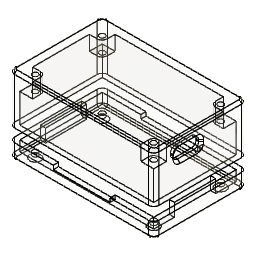
enclosure (Autodesk Fusion 360 design; units mm, degrees)
Autodesk Fusion 360 part; units mm, degrees
sketch "Sketch1" plane through (0, 0, 0) normal (0, 0, 1) x (1, 0, 0) in component "Enclosure-Bottom"
  line L0 (0, 0) -> (50, 0) construction
  line L1 (50, 0) -> (50, 30) construction
  line L2 (50, 30) -> (0, 30) construction
  line L3 (0, 30) -> (0, 0) construction
  line L4 (-1, -1) -> (51, -1)
  line L5 (51, -1) -> (51, 31)
  line L6 (51, 31) -> (-1, 31)
  line L7 (-1, 31) -> (-1, -1)
  line L8 (-1, -3) -> (51, -3)
  line L9 (53, -1) -> (53, 31)
  line L10 (51, 33) -> (-1, 33)
  line L11 (-3, 31) -> (-3, -1)
  arc A0 (53, 31) -> (51, 33) centre (51, 31) ccw
  arc A1 (-1, 33) -> (-3, 31) centre (-1, 31) ccw
  arc A2 (-3, -1) -> (-1, -3) centre (-1, -1) ccw
  arc A3 (51, -3) -> (53, -1) centre (51, -1) ccw
  dimension "d1" = 50
  dimension "d2" = 30
  dimension "d5" = 1
  dimension "d9" = 2
  dimension "d23" = 3
  dimension "d25" = 3
  dimension "d26" = 3
  dimension "d27" = 3
  constraint horizontal L0
  constraint vertical L1
  constraint horizontal L2
  constraint vertical L3
  constraint coincident L0.start L3.end
  constraint parallel L0 L8
  constraint parallel L1 L9
  constraint parallel L2 L10
  constraint parallel L3 L11
  constraint tangent L9 A0
  constraint tangent L10 A0
  constraint tangent L10 A1
  constraint tangent L11 A1
  constraint equal A0 A1
  constraint tangent L11 A2
  constraint tangent L8 A2
  constraint equal A0 A2
  constraint tangent L8 A3
  constraint tangent L9 A3
  constraint equal A0 A3
  measures "d1" distance of L1.end L2.end
  measures "d2" distance of L0.end L1.end
  measures "d9" radius of A0
  measures "d23" distance of L2 L10
  measures "d25" distance of L0 L8
  measures "d26" distance of L3 L11
  measures "d27" distance of L1 L9
extrude "Extrude1" add sketch "Sketch1" against normal blind 2 contours L4 L5 L6 L7 | L8 L9 L10 L11 A0 A1 A2 A3 makes body 1 in component "Enclosure-Bottom"
extrude "Extrude2" add sketch "Sketch1" along normal blind 4 bodies 1 in component "Enclosure-Bottom"
ref_plane "WorkPlane1" through (25, 15, 26) normal (0, 0, 1) x (1, 0, 0)
sketch "Sketch1 (2)" plane through (22.5, 15, 26) normal (0, 0, 1) x (1, 0, 0) in component "Enclosure-Top"
  line L0 (-23.5, -16) -> (28.5, -16)
  line L1 (-23.5, 16) -> (-23.5, -16)
  line L2 (28.5, 16) -> (-23.5, 16)
  line L3 (28.5, -16) -> (28.5, 16)
  line L4 (-23.5, -18) -> (28.5, -18)
  arc A0 (28.5, -18) -> (30.5, -16) centre (28.5, -16) ccw
  line L5 (30.5, -16) -> (30.5, 16)
  line L6 (-25.5, 16) -> (-25.5, -16)
  arc A1 (-25.5, -16) -> (-23.5, -18) centre (-23.5, -16) ccw
  line L7 (28.5, 18) -> (-23.5, 18)
  arc A2 (-23.5, 18) -> (-25.5, 16) centre (-23.5, 16) ccw
  arc A3 (30.5, 16) -> (28.5, 18) centre (28.5, 16) ccw
extrude "Extrude1'" add sketch "Sketch1 (2)" against normal blind 17 separate body makes body 2 in component "Enclosure-Top"
extrude "Extrude2'" add sketch "Sketch1 (2)" along normal blind 2 contours L0 L1 L2 L3 | L4 A0 L5 L6 A1 L7 A2 A3 bodies 2 in component "Enclosure-Top"
fillet "Fillet1" radius 1 8 edges at (53, 15, 28) (52.4142, 32.4142, 28) (25, 33, 28) (-2.4142, 32.4142, 28) (-3, 15, 28) (-2.4142, -2.4142, 28) (25, -3, 28) (52.4142, -2.4142, 28) on bodies 2 in component "Enclosure-Top"
fillet "Fillet1'" radius 1 8 edges at (-3, 15, -2) (-2.4142, 32.4142, -2) (25, 33, -2) (52.4142, 32.4142, -2) (53, 15, -2) (52.4142, -2.4142, -2) (25, -3, -2) (-2.4142, -2.4142, -2) on bodies 1 in component "Enclosure-Bottom"
sketch "Sketch2" plane through (0, 0, 26) normal (0, 0, -1) x (1, 0, 0) in component "Enclosure-Top"
  line L0 (51, 1) -> (-1, 1)
  line L1 (-1, 1) -> (-1, -31)
  line L2 (-1, -31) -> (51, -31)
  line L3 (51, -31) -> (51, 1)
  line L4 (51, -2) -> (-1, -2) construction
  line L5 (2, 1) -> (2, -31) construction
  line L6 (-1, 1) -> (51, 1)
  line L7 (-1, -31) -> (-1, 1)
  line L8 (51, 1) -> (51, -31)
  line L9 (51, -31) -> (-1, -31)
  line L10 (25, 1) -> (25, -31) construction
  line L11 (51, -15) -> (-1, -15) construction
  line L12 (51, -28) -> (-1, -28) construction
  line L13 (48, 1) -> (48, -31) construction
  circle A0 centre (48, -2) radius 1.1
  line L14 (48, -4) -> (51, -4)
  line L15 (46, -2) -> (46, 1)
  arc A1 (46, -2) -> (48, -4) centre (48, -2) ccw
  circle A2 centre (2, -2) radius 1.1
  line L16 (4, -2) -> (4, 1)
  arc A3 (2, -4) -> (4, -2) centre (2, -2) ccw
  line L17 (2, -4) -> (-1, -4)
  circle A4 centre (2, -28) radius 1.1
  line L18 (4, -28) -> (4, -31)
  arc A5 (4, -28) -> (2, -26) centre (2, -28) ccw
  line L19 (2, -26) -> (-1, -26)
  line L20 (48, -26) -> (51, -26)
  circle A6 centre (48, -28) radius 1.1
  arc A7 (48, -26) -> (46, -28) centre (48, -28) ccw
  line L21 (46, -28) -> (46, -31)
  dimension "d28" = 3
  dimension "d29" = 3
  dimension "d30" = 2.2
  dimension "d31" = 4
  constraint coincident L3 L4.start
  constraint coincident L1 L4.end
  constraint perpendicular L1 L4
  constraint coincident L0 L5.start
  constraint coincident L2 L5.end
  constraint perpendicular L2 L5
  constraint midpoint L6 L10.start
  constraint midpoint L9 L10.end
  constraint midpoint L8 L11.start
  constraint midpoint L7 L11.end
  constraint symmetric L4.start L11 L12.start
  constraint symmetric L4.end L11 L12.end
  constraint symmetric L5.start L10 L13.start
  constraint symmetric L5.end L10 L13.end
  constraint coincident L13 A0.centre
  constraint coincident L4 A0.centre
  constraint concentric A0 A1
  constraint coincident L13 L14.start
  constraint coincident L8 L14.end
  constraint tangent L14 A1
  constraint coincident L4 L15.start
  constraint coincident L6 L15.end
  constraint tangent L15 A1
  constraint symmetric L10 A0 A2
  constraint symmetric L10 L14.start A3.start
  constraint symmetric L10 L14.end L17.end
  constraint symmetric L10 L15.start L16.start
  constraint symmetric L10 L15.end L16.end
  constraint symmetric L10 A1 A3
  constraint symmetric L11 A0 A6
  constraint symmetric L11 L14.start L20.start
  constraint symmetric L11 L14.end L20.end
  constraint symmetric L11 L15.start A7.end
  constraint symmetric L11 L15.end L21.end
  constraint symmetric L11 A1 A7
  constraint symmetric L11 A2 A4
  constraint symmetric L11 L16.start L18.start
  constraint symmetric L11 L16.end L18.end
  constraint symmetric L11 A3.start A5.end
  constraint symmetric L11 A3 A5
  constraint symmetric L11 L17.end L19.end
  measures "d28" distance of L0 L4
  measures "d29" distance of L5 L7
  measures "d30" diameter of A0
  measures "d31" diameter of A1
extrude "Extrude3" add sketch "Sketch2" along normal blind 5.7143 contours L0 L3 L6 L8 L14 L15 A1 | L0 L1 L6 L7 L16 A3 L17 | L2 L3 L8 L9 L20 A7 L21 | L1 L2 L7 L9 L18 A5 L19 bodies 2 in component "Enclosure-Top"
sketch "Sketch2 (2)" plane through (0, 0, 0) normal (0, 0, 1) x (-1, 0, 0) in component "Enclosure-Bottom"
  line L0 (1, 1) -> (-51, 1)
  line L1 (-51, 1) -> (-51, -31)
  line L2 (-51, -31) -> (1, -31)
  line L3 (1, -31) -> (1, 1)
  line L4 (1, -31) -> (-51, -31)
  line L5 (-51, -31) -> (-51, 1)
  line L6 (1, 1) -> (1, -31)
  line L7 (-51, 1) -> (1, 1)
  line L8 (-25, -31) -> (-25, 1) construction
  line L9 (-51, -15) -> (1, -15) construction
  line L10 (-49, -23) -> (-51, -23)
  line L11 (-51, -23) -> (-51, -7)
  line L12 (-51, -7) -> (-49, -7)
  line L13 (-49, -7) -> (-49, -23)
  line L14 (-1, -7) -> (-1, -23)
  line L15 (-1, -23) -> (1, -23)
  line L16 (1, -7) -> (-1, -7)
  dimension "d44" = 2
  dimension "d45" = 16
  dimension "d46" = 8
  constraint midpoint L4 L8.start
  constraint midpoint L7 L8.end
  constraint midpoint L5 L9.start
  constraint midpoint L6 L9.end
  constraint horizontal L10
  constraint vertical L11
  constraint horizontal L12
  constraint vertical L13
  constraint coincident L0.end L11
  constraint symmetric L8 L10.start L14.end
  constraint symmetric L8 L10.end L15.end
  constraint symmetric L8 L11.end L16.start
  constraint symmetric L8 L12.end L14.start
  measures "d44" distance of L10.start L10.end
  measures "d45" distance of L10.start L12.end
  measures "d46" distance of L9 L10
extrude "Extrude3'" add sketch "Sketch2 (2)" along normal blind 5 contours L3 L6 L14 L15 L16 | L1 L5 L10 L11 L12 L13 bodies 1 in component "Enclosure-Bottom"
sketch "Sketch4" plane through (0, 0, -2) normal (0, 0, -1) x (1, 0, 0) in component "Enclosure-Bottom"
  line L0 (-2, 1) -> (-2, -31)
  arc A0 (-2, -31) -> (-1, -32) centre (-1, -31) ccw
  line L1 (-1, -32) -> (51, -32)
  arc A1 (51, -32) -> (52, -31) centre (51, -31) ccw
  line L2 (52, -31) -> (52, 1)
  arc A2 (52, 1) -> (51, 2) centre (51, 1) ccw
  line L3 (51, 2) -> (-1, 2)
  arc A3 (-1, 2) -> (-2, 1) centre (-1, 1) ccw
  circle A4 centre (48, -2) radius 1.1
  circle A5 centre (2, -2) radius 1.1
  circle A6 centre (2, -28) radius 1.1
  circle A7 centre (48, -28) radius 1.1
extrude "Extrude4" cut sketch "Sketch4" against normal up to surface (2 mm away) contours A4 | A5 | A6 | A7 bodies 1 in component "Enclosure-Bottom"
chamfer "Chamfer1" distance 1 angle 45 4 edges at (0.9744, 27.6022, -2) (46.9744, 27.6022, -2) (46.9744, 1.6022, -2) (0.9744, 1.6022, -2) on bodies 1 in component "Enclosure-Bottom"
sketch "Sketch5" plane through (0, 0, 4) normal (0, 0, 1) x (-1, 0, 0) in component "Enclosure-Bottom"
  line L0 (1, 1) -> (1, -7)
  line L1 (1, -7) -> (1, -23)
  line L2 (1, -23) -> (1, -31)
  line L3 (1, -31) -> (-51, -31)
  line L4 (-51, -31) -> (-51, -23)
  line L5 (-51, -23) -> (-51, -7)
  line L6 (-51, -7) -> (-51, 1)
  line L7 (-51, 1) -> (1, 1) construction
  arc A0 (-51, 3) -> (-53, 1) centre (-51, 1) ccw
  line L8 (-53, 1) -> (-53, -31)
  arc A1 (-53, -31) -> (-51, -33) centre (-51, -31) ccw
  line L9 (-51, -33) -> (1, -33)
  arc A2 (1, -33) -> (3, -31) centre (1, -31) ccw
  line L10 (3, -31) -> (3, 1)
  arc A3 (3, 1) -> (1, 3) centre (1, 1) ccw
  line L11 (1, 3) -> (-51, 3)
  line L12 (1, -31) -> (-51, -31) construction
  line L13 (-51, 1) -> (1, 1)
  line L14 (-25, -31) -> (-25, 1) construction
  line L15 (-51, -15) -> (0, -15) construction
  line L16 (-14, -33) -> (-36, -33)
  line L17 (-36, -33) -> (-36, -31)
  line L18 (-36, -31) -> (-14, -31)
  line L19 (-14, -31) -> (-14, -33)
  line L20 (-14, 1) -> (-14, 3)
  line L21 (-14, 3) -> (-36, 3)
  line L22 (-36, 1) -> (-14, 1)
  line L23 (-36, 3) -> (-36, 1)
  dimension "d50" = 22
  dimension "d51" = 2
  dimension "d52" = 11
  constraint midpoint L12 L14.start
  constraint midpoint L13 L14.end
  constraint midpoint L5 L15.start
  constraint perpendicular L1 L15
  constraint horizontal L16
  constraint vertical L17
  constraint horizontal L18
  constraint vertical L19
  constraint coincident L3.end L18
  constraint symmetric L15 L16.start L20.end
  constraint symmetric L15 L16.end L21.end
  constraint symmetric L15 L17.end L22.start
  constraint symmetric L15 L18.end L20.start
  measures "d50" distance of L17.end L18.end
  measures "d51" distance of L16.start L18.end
  measures "d52" distance of L14 L17
extrude "Extrude5" cut sketch "Sketch5" against normal blind 1.5 contours L11 L13 L20 L21 L22 L23 | L3 L9 L16 L17 L18 L19 bodies 1 in component "Enclosure-Bottom"
sketch "Sketch3" plane through (53, 0, 0) normal (1, 0, 0) x (0, 1, 0) in component "Enclosure-Top"
  line L0 (31, 27) -> (-1, 27)
  line L1 (-1, 27) -> (-1, 9)
  line L2 (-1, 9) -> (31, 9)
  line L3 (31, 9) -> (31, 27)
  line L4 (9.99, 19.9857) -> (13.63, 19.9857)
  arc A0 (13.63, 19.9857) -> (15.41, 21.7657) centre (13.63, 21.7657) ccw
  line L5 (15.41, 21.7657) -> (15.41, 22.3657)
  arc A1 (15.41, 22.3657) -> (13.63, 24.1457) centre (13.63, 22.3657) ccw
  line L6 (13.63, 24.1457) -> (7.25, 24.1457)
  arc A2 (7.25, 24.1457) -> (5.47, 22.3657) centre (7.25, 22.3657) ccw
  line L7 (5.47, 22.3657) -> (5.47, 21.7657)
  arc A3 (5.47, 21.7657) -> (7.25, 19.9857) centre (7.25, 21.7657) ccw
  line L8 (7.25, 19.9857) -> (9.94, 19.9857)
  line L9 (9.99, 19.9857) -> (9.94, 19.9857)
  constraint parallel L8 L9
  constraint tangent L5 A1
  constraint tangent A2 L7
  constraint tangent L4 A0
  constraint tangent A0 L5
  constraint tangent L7 A3
  constraint tangent A1 L6
  constraint tangent L6 A2
  constraint tangent A3 L8
extrude "Extrude4'" cut sketch "Sketch3" against normal up to surface (2 mm away) contours L4 A0 L5 A1 L6 A2 L7 A3 L8 L9 bodies 2 in component "Enclosure-Top"
chamfer "Chamfer1'" distance 1 angle 45 8 edges at (53, 14.8887, 23.6244) (53, 15.41, 22.0657) (53, 14.8887, 20.5071) (53, 10.44, 19.9857) (53, 5.9913, 20.5071) (53, 5.47, 22.0657) (53, 5.9913, 23.6244) (53, 10.44, 24.1457) on bodies 2 in component "Enclosure-Top"
component "Enclosure-Bottom" placed x (1, 0, 0) y (0, 1, 0) z (0, 0, 1) at (0, 0, 0)
component "Enclosure-Top" placed x (1, 0, 0) y (0, 1, 0) z (0, 0, 1) at (0, 0, 0)
equation "d1 = length"
equation "d2 = width"
equation "wall_thickness = 2 mm"
equation "margin = 1 mm"
equation "d5 = margin"
equation "fillet_radius = 2 mm"
equation "height = 20 mm"
equation "d9 = fillet_radius"
equation "d10 = -wall_thickness"
equation "d12 = height / 5"
equation "d14 = height + wall_thickness"
equation "d15 = -height * 0.85"
equation "d17 = wall_thickness"
equation "d20 = 0.5 * fillet_radius"
equation "d22 = 0.5 * fillet_radius"
equation "d23 = wall_thickness + margin"
equation "d25 = wall_thickness + margin"
equation "d26 = wall_thickness + margin"
equation "d27 = wall_thickness + margin"
equation "d28 = 2 mm + margin"
equation "d29 = 2 mm + margin"
equation "d32 = height / 3.5"
equation "d37 = height / 4"
equation "length = 50 mm"
equation "width = 30 mm"
equation "d44 = wall_thickness"
equation "d45 = wall_thickness * 8"
equation "d46 = ( wall_thickness * 4 )"
equation "d51 = wall_thickness"
